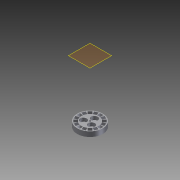
# Autodesk Inventor part: Bottom4
Saved by Autodesk Inventor 2012 (Build 160160000, 160)
## iProperties
Created: 2015-08-07
Part Number: Bottom4
Material: Default
Document SubType Name: Modeling
Designer: Craig
Density: 1 g/cm^3
Autodesk Inventor part; units mm, degrees
(part 1 of 3)
ref_plane "YZ Plane" through (0, 0, 0) normal (1, 0, 0) x (0, 1, 0)
ref_plane "XZ Plane" through (0, 0, 0) normal (0, 1, 0) x (-1, 0, 0)
ref_plane "XY Plane" through (0, 0, 0) normal (0, 0, 1) x (1, 0, 0)
sketch "BOTTOM" plane through (0, 0, 0) normal (0, 0, 1) x (1, 0, 0)
  line L0 (59.975, -52.845) -> (63.225, -52.845)
  line L1 (63.225, -52.845) -> (63.225, -49.595)
  line L2 (63.225, -49.595) -> (59.975, -49.595)
  line L3 (59.975, -49.595) -> (59.975, -52.845)
  line L4 (0, 0) -> (1, 0)
  line L5 (49.6005, -59.9784) -> (49.5995, -63.2284)
  line L6 (49.5995, -63.2284) -> (52.8495, -63.2295)
  line L7 (52.8495, -63.2295) -> (52.8505, -59.9795)
  line L8 (52.8505, -59.9795) -> (49.6005, -59.9784)
  line L9 (0, 0) -> (1, 0)
  line L10 (49.8915, -64.6991) -> (51.1369, -67.701)
  line L11 (51.1369, -67.701) -> (54.1388, -66.4556)
  line L12 (54.1388, -66.4556) -> (52.8934, -63.4537)
  line L13 (52.8934, -63.4537) -> (49.8915, -64.6991)
  line L14 (0, 0) -> (1, 0)
  line L15 (51.9695, -68.9456) -> (54.2706, -71.2407)
  line L16 (54.2706, -71.2407) -> (56.5657, -68.9397)
  line L17 (56.5657, -68.9397) -> (54.2646, -66.6445)
  line L18 (54.2646, -66.6445) -> (51.9695, -68.9456)
  line L19 (0, 0) -> (1, 0)
  line L20 (55.5107, -72.0693) -> (58.514, -73.3112)
  line L21 (58.514, -73.3112) -> (59.756, -70.3079)
  line L22 (59.756, -70.3079) -> (56.7527, -69.0659)
  line L23 (56.7527, -69.0659) -> (55.5107, -72.0693)
  line L24 (0, 0) -> (1, 0)
  line L25 (59.9813, -73.6029) -> (63.2313, -73.6008)
  line L26 (63.2313, -73.6008) -> (63.2293, -70.3508)
  line L27 (63.2293, -70.3508) -> (59.9793, -70.3529)
  line L28 (59.9793, -70.3529) -> (59.9813, -73.6029)
  line L29 (0, 0) -> (1, 0)
  line L30 (64.6994, -73.3084) -> (67.7011, -72.0624)
  line L31 (67.7011, -72.0624) -> (66.455, -69.0607)
  line L32 (66.455, -69.0607) -> (63.4534, -70.3067)
  line L33 (63.4534, -70.3067) -> (64.6994, -73.3084)
  line L34 (0, 0) -> (1, 0)
  line L35 (68.9435, -71.2317) -> (71.24, -68.932)
  line L36 (71.24, -68.932) -> (68.9403, -66.6355)
  line L37 (68.9403, -66.6355) -> (66.6438, -68.9351)
  line L38 (66.6438, -68.9351) -> (68.9435, -71.2317)
  line L39 (0, 0) -> (1, 0)
  line L40 (72.0699, -67.6893) -> (73.3118, -64.686)
  line L41 (73.3118, -64.686) -> (70.3085, -63.4441)
  line L42 (70.3085, -63.4441) -> (69.0665, -66.4474)
  line L43 (69.0665, -66.4474) -> (72.0699, -67.6893)
  line L44 (0, 0) -> (1, 0)
  line L45 (73.6037, -63.2169) -> (73.6013, -59.9669)
  line L46 (73.6013, -59.9669) -> (70.3513, -59.9694)
  line L47 (70.3513, -59.9694) -> (70.3537, -63.2194)
  line L48 (70.3537, -63.2194) -> (73.6037, -63.2169)
  line L49 (0, 0) -> (1, 0)
  line L50 (73.3095, -58.5022) -> (72.0634, -55.5006)
  line L51 (72.0634, -55.5006) -> (69.0618, -56.7467)
  line L52 (69.0618, -56.7467) -> (70.3079, -59.7483)
  line L53 (70.3079, -59.7483) -> (73.3095, -58.5022)
  line L54 (0, 0) -> (1, 0)
  line L55 (71.2319, -54.2571) -> (68.932, -51.9607)
  line L56 (68.932, -51.9607) -> (66.6357, -54.2606)
  line L57 (66.6357, -54.2606) -> (68.9355, -56.5569)
  line L58 (68.9355, -56.5569) -> (71.2319, -54.2571)
  line L59 (0, 0) -> (1, 0)
  line L60 (67.6871, -51.1295) -> (64.6835, -49.8882)
  line L61 (64.6835, -49.8882) -> (63.4422, -52.8918)
  line L62 (63.4422, -52.8918) -> (66.4458, -54.1331)
  line L63 (66.4458, -54.1331) -> (67.6871, -51.1295)
  line L64 (0, 0) -> (1, 0)
  line L65 (58.5019, -49.891) -> (55.5, -51.1366)
  line L66 (55.5, -51.1366) -> (56.7456, -54.1384)
  line L67 (56.7456, -54.1384) -> (59.7474, -52.8928)
  line L68 (59.7474, -52.8928) -> (58.5019, -49.891)
  line L69 (0, 0) -> (1, 0)
  line L70 (54.2559, -51.9683) -> (51.9595, -54.2681)
  line L71 (51.9595, -54.2681) -> (54.2593, -56.5645)
  line L72 (54.2593, -56.5645) -> (56.5557, -54.2647)
  line L73 (56.5557, -54.2647) -> (54.2559, -51.9683)
  line L74 (0, 0) -> (1, 0)
  line L75 (51.1301, -55.5101) -> (49.8882, -58.5135)
  line L76 (49.8882, -58.5135) -> (52.8916, -59.7554)
  line L77 (52.8916, -59.7554) -> (54.1334, -56.752)
  line L78 (54.1334, -56.752) -> (51.1301, -55.5101)
  line L79 (0, 0) -> (1, 0)
  arc A0 (48.6, -61.6029) -> (52.9038, -71.2653) centre (61.5843, -61.6091) ccw
  arc A1 (52.9038, -71.2653) -> (72.8082, -68.1903) centre (61.6004, -61.5999) ccw
  arc A2 (72.8082, -68.1903) -> (74.163, -58.2471) centre (61.5989, -61.5991) ccw
  arc A3 (74.163, -58.2471) -> (59.1805, -48.8249) centre (61.5986, -61.6031) ccw
  arc A4 (59.1805, -48.8249) -> (48.8055, -59.2842) centre (61.5989, -61.5991) ccw
  arc A5 (48.8055, -59.2842) -> (48.6, -61.6029) centre (61.5557, -61.583) ccw
  line L80 (0, 0) -> (1, 0)
  line L81 (55.9748, -59.9753) -> (56.0584, -59.9774)
  line L82 (56.0584, -59.9774) -> (56.141, -59.9837)
  line L83 (56.141, -59.9837) -> (56.2223, -59.994)
  line L84 (56.2223, -59.994) -> (56.3023, -60.0083)
  line L85 (56.3023, -60.0083) -> (56.3809, -60.0264)
  line L86 (56.3809, -60.0264) -> (56.458, -60.0483)
  line L87 (56.458, -60.0483) -> (56.5335, -60.0738)
  line L88 (56.5335, -60.0738) -> (56.6073, -60.1029)
  line L89 (56.6073, -60.1029) -> (56.6793, -60.1354)
  line L90 (56.6793, -60.1354) -> (56.7494, -60.1713)
  line L91 (56.7494, -60.1713) -> (56.8175, -60.2104)
  line L92 (56.8175, -60.2104) -> (56.8834, -60.2527)
  line L93 (56.8834, -60.2527) -> (56.9471, -60.298)
  line L94 (56.9471, -60.298) -> (57.0085, -60.3462)
  line L95 (57.0085, -60.3462) -> (57.0675, -60.3973)
  line L96 (57.0675, -60.3973) -> (57.1239, -60.4511)
  line L97 (57.1239, -60.4511) -> (57.1777, -60.5075)
  line L98 (57.1777, -60.5075) -> (57.2288, -60.5665)
  line L99 (57.2288, -60.5665) -> (57.2771, -60.6279)
  line L100 (57.2771, -60.6279) -> (57.3224, -60.6916)
  line L101 (57.3224, -60.6916) -> (57.3646, -60.7575)
  line L102 (57.3646, -60.7575) -> (57.4038, -60.8255)
  line L103 (57.4038, -60.8255) -> (57.4397, -60.8956)
  line L104 (57.4397, -60.8956) -> (57.4722, -60.9676)
  line L105 (57.4722, -60.9676) -> (57.5013, -61.0414)
  line L106 (57.5013, -61.0414) -> (57.5269, -61.1169)
  line L107 (57.5269, -61.1169) -> (57.5488, -61.194)
  line L108 (57.5488, -61.194) -> (57.5669, -61.2726)
  line L109 (57.5669, -61.2726) -> (57.5812, -61.3526)
  line L110 (57.5812, -61.3526) -> (57.5916, -61.4339)
  line L111 (57.5916, -61.4339) -> (57.5979, -61.5165)
  line L112 (57.5979, -61.5165) -> (57.6, -61.6001)
  line L113 (57.6, -61.6001) -> (57.5979, -61.6837)
  line L114 (57.5979, -61.6837) -> (57.5916, -61.7662)
  line L115 (57.5916, -61.7662) -> (57.5813, -61.8476)
  line L116 (57.5813, -61.8476) -> (57.567, -61.9276)
  line L117 (57.567, -61.9276) -> (57.5489, -62.0062)
  line L118 (57.5489, -62.0062) -> (57.527, -62.0833)
  line L119 (57.527, -62.0833) -> (57.5015, -62.1588)
  line L120 (57.5015, -62.1588) -> (57.4724, -62.2326)
  line L121 (57.4724, -62.2326) -> (57.4398, -62.3046)
  line L122 (57.4398, -62.3046) -> (57.404, -62.3747)
  line L123 (57.404, -62.3747) -> (57.3648, -62.4427)
  line L124 (57.3648, -62.4427) -> (57.3226, -62.5087)
  line L125 (57.3226, -62.5087) -> (57.2773, -62.5724)
  line L126 (57.2773, -62.5724) -> (57.2291, -62.6338)
  line L127 (57.2291, -62.6338) -> (57.178, -62.6928)
  line L128 (57.178, -62.6928) -> (57.1242, -62.7492)
  line L129 (57.1242, -62.7492) -> (57.0678, -62.803)
  line L130 (57.0678, -62.803) -> (57.0088, -62.8541)
  line L131 (57.0088, -62.8541) -> (56.9474, -62.9023)
  line L132 (56.9474, -62.9023) -> (56.8837, -62.9476)
  line L133 (56.8837, -62.9476) -> (56.8178, -62.9899)
  line L134 (56.8178, -62.9899) -> (56.7497, -63.0291)
  line L135 (56.7497, -63.0291) -> (56.6797, -63.065)
  line L136 (56.6797, -63.065) -> (56.6077, -63.0975)
  line L137 (56.6077, -63.0975) -> (56.5339, -63.1266)
  line L138 (56.5339, -63.1266) -> (56.4584, -63.1522)
  line L139 (56.4584, -63.1522) -> (56.3813, -63.1741)
  line L140 (56.3813, -63.1741) -> (56.3027, -63.1922)
  line L141 (56.3027, -63.1922) -> (56.2227, -63.2065)
  line L142 (56.2227, -63.2065) -> (56.1413, -63.2169)
  line L143 (56.1413, -63.2169) -> (56.0588, -63.2232)
  line L144 (56.0588, -63.2232) -> (55.9752, -63.2253)
  line L145 (55.9752, -63.2253) -> (55.8916, -63.2232)
  line L146 (55.8916, -63.2232) -> (55.809, -63.2169)
  line L147 (55.809, -63.2169) -> (55.7277, -63.2066)
  line L148 (55.7277, -63.2066) -> (55.6477, -63.1923)
  line L149 (55.6477, -63.1923) -> (55.5691, -63.1742)
  line L150 (55.5691, -63.1742) -> (55.492, -63.1523)
  line L151 (55.492, -63.1523) -> (55.4165, -63.1267)
  line L152 (55.4165, -63.1267) -> (55.3427, -63.0977)
  line L153 (55.3427, -63.0977) -> (55.2707, -63.0651)
  line L154 (55.2707, -63.0651) -> (55.2006, -63.0292)
  line L155 (55.2006, -63.0292) -> (55.1325, -62.9901)
  line L156 (55.1325, -62.9901) -> (55.0666, -62.9479)
  line L157 (55.0666, -62.9479) -> (55.0029, -62.9026)
  line L158 (55.0029, -62.9026) -> (54.9415, -62.8543)
  line L159 (54.9415, -62.8543) -> (54.8825, -62.8033)
  line L160 (54.8825, -62.8033) -> (54.8261, -62.7495)
  line L161 (54.8261, -62.7495) -> (54.7723, -62.693)
  line L162 (54.7723, -62.693) -> (54.7212, -62.6341)
  line L163 (54.7212, -62.6341) -> (54.6729, -62.5727)
  line L164 (54.6729, -62.5727) -> (54.6276, -62.509)
  line L165 (54.6276, -62.509) -> (54.5854, -62.4431)
  line L166 (54.5854, -62.4431) -> (54.5462, -62.375)
  line L167 (54.5462, -62.375) -> (54.5103, -62.305)
  line L168 (54.5103, -62.305) -> (54.4778, -62.233)
  line L169 (54.4778, -62.233) -> (54.4487, -62.1592)
  line L170 (54.4487, -62.1592) -> (54.4231, -62.0837)
  line L171 (54.4231, -62.0837) -> (54.4012, -62.0066)
  line L172 (54.4012, -62.0066) -> (54.3831, -61.928)
  line L173 (54.3831, -61.928) -> (54.3688, -61.8479)
  line L174 (54.3688, -61.8479) -> (54.3584, -61.7666)
  line L175 (54.3584, -61.7666) -> (54.3521, -61.6841)
  line L176 (54.3521, -61.6841) -> (54.35, -61.6005)
  line L177 (54.35, -61.6005) -> (54.3521, -61.5169)
  line L178 (54.3521, -61.5169) -> (54.3584, -61.4343)
  line L179 (54.3584, -61.4343) -> (54.3687, -61.353)
  line L180 (54.3687, -61.353) -> (54.383, -61.273)
  line L181 (54.383, -61.273) -> (54.4011, -61.1944)
  line L182 (54.4011, -61.1944) -> (54.423, -61.1172)
  line L183 (54.423, -61.1172) -> (54.4485, -61.0417)
  line L184 (54.4485, -61.0417) -> (54.4776, -60.9679)
  line L185 (54.4776, -60.9679) -> (54.5102, -60.8959)
  line L186 (54.5102, -60.8959) -> (54.546, -60.8259)
  line L187 (54.546, -60.8259) -> (54.5852, -60.7578)
  line L188 (54.5852, -60.7578) -> (54.6274, -60.6919)
  line L189 (54.6274, -60.6919) -> (54.6727, -60.6282)
  line L190 (54.6727, -60.6282) -> (54.7209, -60.5668)
  line L191 (54.7209, -60.5668) -> (54.772, -60.5078)
  line L192 (54.772, -60.5078) -> (54.8258, -60.4514)
  line L193 (54.8258, -60.4514) -> (54.8822, -60.3976)
  line L194 (54.8822, -60.3976) -> (54.9412, -60.3465)
  line L195 (54.9412, -60.3465) -> (55.0026, -60.2982)
  line L196 (55.0026, -60.2982) -> (55.0663, -60.2529)
  line L197 (55.0663, -60.2529) -> (55.1322, -60.2106)
  line L198 (55.1322, -60.2106) -> (55.2003, -60.1715)
  line L199 (55.2003, -60.1715) -> (55.2703, -60.1356)
  line L200 (55.2703, -60.1356) -> (55.3423, -60.1031)
  line L201 (55.3423, -60.1031) -> (55.4161, -60.074)
  line L202 (55.4161, -60.074) -> (55.4916, -60.0484)
  line L203 (55.4916, -60.0484) -> (55.5687, -60.0265)
  line L204 (55.5687, -60.0265) -> (55.6473, -60.0083)
  line L205 (55.6473, -60.0083) -> (55.7273, -59.994)
  line L206 (55.7273, -59.994) -> (55.8087, -59.9837)
  line L207 (55.8087, -59.9837) -> (55.8912, -59.9774)
  line L208 (55.8912, -59.9774) -> (55.9748, -59.9753)
  line L209 (0, 0) -> (1, 0)
  line L210 (59.977, -67.2264) -> (59.9791, -67.1428)
  line L211 (59.9791, -67.1428) -> (59.9853, -67.0602)
  line L212 (59.9853, -67.0602) -> (59.9956, -66.9789)
  line L213 (59.9956, -66.9789) -> (60.0099, -66.8989)
  line L214 (60.0099, -66.8989) -> (60.028, -66.8202)
  line L215 (60.028, -66.8202) -> (60.0498, -66.7431)
  line L216 (60.0498, -66.7431) -> (60.0754, -66.6676)
  line L217 (60.0754, -66.6676) -> (60.1044, -66.5938)
  line L218 (60.1044, -66.5938) -> (60.1369, -66.5218)
  line L219 (60.1369, -66.5218) -> (60.1728, -66.4517)
  line L220 (60.1728, -66.4517) -> (60.2119, -66.3837)
  line L221 (60.2119, -66.3837) -> (60.2541, -66.3177)
  line L222 (60.2541, -66.3177) -> (60.2994, -66.254)
  line L223 (60.2994, -66.254) -> (60.3476, -66.1926)
  line L224 (60.3476, -66.1926) -> (60.3987, -66.1336)
  line L225 (60.3987, -66.1336) -> (60.4524, -66.0771)
  line L226 (60.4524, -66.0771) -> (60.5088, -66.0233)
  line L227 (60.5088, -66.0233) -> (60.5678, -65.9722)
  line L228 (60.5678, -65.9722) -> (60.6291, -65.9239)
  line L229 (60.6291, -65.9239) -> (60.6928, -65.8786)
  line L230 (60.6928, -65.8786) -> (60.7587, -65.8363)
  line L231 (60.7587, -65.8363) -> (60.8268, -65.7971)
  line L232 (60.8268, -65.7971) -> (60.8968, -65.7612)
  line L233 (60.8968, -65.7612) -> (60.9688, -65.7286)
  line L234 (60.9688, -65.7286) -> (61.0426, -65.6995)
  line L235 (61.0426, -65.6995) -> (61.1181, -65.6739)
  line L236 (61.1181, -65.6739) -> (61.1952, -65.652)
  line L237 (61.1952, -65.652) -> (61.2738, -65.6338)
  line L238 (61.2738, -65.6338) -> (61.3538, -65.6195)
  line L239 (61.3538, -65.6195) -> (61.4351, -65.6091)
  line L240 (61.4351, -65.6091) -> (61.5176, -65.6028)
  line L241 (61.5176, -65.6028) -> (61.6013, -65.6006)
  line L242 (61.6013, -65.6006) -> (61.6849, -65.6027)
  line L243 (61.6849, -65.6027) -> (61.7674, -65.609)
  line L244 (61.7674, -65.609) -> (61.8487, -65.6193)
  line L245 (61.8487, -65.6193) -> (61.9288, -65.6335)
  line L246 (61.9288, -65.6335) -> (62.0074, -65.6516)
  line L247 (62.0074, -65.6516) -> (62.0845, -65.6735)
  line L248 (62.0845, -65.6735) -> (62.16, -65.699)
  line L249 (62.16, -65.699) -> (62.2338, -65.7281)
  line L250 (62.2338, -65.7281) -> (62.3058, -65.7606)
  line L251 (62.3058, -65.7606) -> (62.3759, -65.7964)
  line L252 (62.3759, -65.7964) -> (62.444, -65.8355)
  line L253 (62.444, -65.8355) -> (62.5099, -65.8777)
  line L254 (62.5099, -65.8777) -> (62.5737, -65.923)
  line L255 (62.5737, -65.923) -> (62.6351, -65.9712)
  line L256 (62.6351, -65.9712) -> (62.6941, -66.0223)
  line L257 (62.6941, -66.0223) -> (62.7505, -66.0761)
  line L258 (62.7505, -66.0761) -> (62.8044, -66.1325)
  line L259 (62.8044, -66.1325) -> (62.8555, -66.1914)
  line L260 (62.8555, -66.1914) -> (62.9037, -66.2528)
  line L261 (62.9037, -66.2528) -> (62.9491, -66.3165)
  line L262 (62.9491, -66.3165) -> (62.9914, -66.3824)
  line L263 (62.9914, -66.3824) -> (63.0305, -66.4504)
  line L264 (63.0305, -66.4504) -> (63.0664, -66.5205)
  line L265 (63.0664, -66.5205) -> (63.099, -66.5924)
  line L266 (63.099, -66.5924) -> (63.1281, -66.6662)
  line L267 (63.1281, -66.6662) -> (63.1537, -66.7417)
  line L268 (63.1537, -66.7417) -> (63.1757, -66.8188)
  line L269 (63.1757, -66.8188) -> (63.1938, -66.8974)
  line L270 (63.1938, -66.8974) -> (63.2082, -66.9774)
  line L271 (63.2082, -66.9774) -> (63.2185, -67.0588)
  line L272 (63.2185, -67.0588) -> (63.2249, -67.1413)
  line L273 (63.2249, -67.1413) -> (63.227, -67.2249)
  line L274 (63.227, -67.2249) -> (63.2249, -67.3085)
  line L275 (63.2249, -67.3085) -> (63.2187, -67.391)
  line L276 (63.2187, -67.391) -> (63.2084, -67.4724)
  line L277 (63.2084, -67.4724) -> (63.1941, -67.5524)
  line L278 (63.1941, -67.5524) -> (63.176, -67.631)
  line L279 (63.176, -67.631) -> (63.1542, -67.7082)
  line L280 (63.1542, -67.7082) -> (63.1287, -67.7837)
  line L281 (63.1287, -67.7837) -> (63.0996, -67.8575)
  line L282 (63.0996, -67.8575) -> (63.0671, -67.9295)
  line L283 (63.0671, -67.9295) -> (63.0312, -67.9996)
  line L284 (63.0312, -67.9996) -> (62.9921, -68.0676)
  line L285 (62.9921, -68.0676) -> (62.9499, -68.1336)
  line L286 (62.9499, -68.1336) -> (62.9046, -68.1973)
  line L287 (62.9046, -68.1973) -> (62.8564, -68.2587)
  line L288 (62.8564, -68.2587) -> (62.8054, -68.3177)
  line L289 (62.8054, -68.3177) -> (62.7516, -68.3742)
  line L290 (62.7516, -68.3742) -> (62.6952, -68.428)
  line L291 (62.6952, -68.428) -> (62.6362, -68.4791)
  line L292 (62.6362, -68.4791) -> (62.5749, -68.5274)
  line L293 (62.5749, -68.5274) -> (62.5112, -68.5727)
  line L294 (62.5112, -68.5727) -> (62.4453, -68.615)
  line L295 (62.4453, -68.615) -> (62.3772, -68.6542)
  line L296 (62.3772, -68.6542) -> (62.3072, -68.6901)
  line L297 (62.3072, -68.6901) -> (62.2352, -68.7226)
  line L298 (62.2352, -68.7226) -> (62.1614, -68.7518)
  line L299 (62.1614, -68.7518) -> (62.0859, -68.7774)
  line L300 (62.0859, -68.7774) -> (62.0088, -68.7993)
  line L301 (62.0088, -68.7993) -> (61.9302, -68.8175)
  line L302 (61.9302, -68.8175) -> (61.8502, -68.8318)
  line L303 (61.8502, -68.8318) -> (61.7689, -68.8422)
  line L304 (61.7689, -68.8422) -> (61.6864, -68.8485)
  line L305 (61.6864, -68.8485) -> (61.6028, -68.8506)
  line L306 (61.6028, -68.8506) -> (61.5191, -68.8486)
  line L307 (61.5191, -68.8486) -> (61.4366, -68.8423)
  line L308 (61.4366, -68.8423) -> (61.3553, -68.832)
  line L309 (61.3553, -68.832) -> (61.2752, -68.8178)
  line L310 (61.2752, -68.8178) -> (61.1966, -68.7997)
  line L311 (61.1966, -68.7997) -> (61.1195, -68.7778)
  line L312 (61.1195, -68.7778) -> (61.044, -68.7523)
  line L313 (61.044, -68.7523) -> (60.9702, -68.7232)
  line L314 (60.9702, -68.7232) -> (60.8982, -68.6907)
  line L315 (60.8982, -68.6907) -> (60.8281, -68.6549)
  line L316 (60.8281, -68.6549) -> (60.76, -68.6158)
  line L317 (60.76, -68.6158) -> (60.6941, -68.5735)
  line L318 (60.6941, -68.5735) -> (60.6303, -68.5283)
  line L319 (60.6303, -68.5283) -> (60.5689, -68.48)
  line L320 (60.5689, -68.48) -> (60.5099, -68.429)
  line L321 (60.5099, -68.429) -> (60.4535, -68.3752)
  line L322 (60.4535, -68.3752) -> (60.3997, -68.3188)
  line L323 (60.3997, -68.3188) -> (60.3486, -68.2599)
  line L324 (60.3486, -68.2599) -> (60.3003, -68.1985)
  line L325 (60.3003, -68.1985) -> (60.2549, -68.1348)
  line L326 (60.2549, -68.1348) -> (60.2126, -68.0689)
  line L327 (60.2126, -68.0689) -> (60.1735, -68.0009)
  line L328 (60.1735, -68.0009) -> (60.1376, -67.9308)
  line L329 (60.1376, -67.9308) -> (60.105, -67.8588)
  line L330 (60.105, -67.8588) -> (60.0759, -67.7851)
  line L331 (60.0759, -67.7851) -> (60.0503, -67.7096)
  line L332 (60.0503, -67.7096) -> (60.0284, -67.6325)
  line L333 (60.0284, -67.6325) -> (60.0102, -67.5539)
  line L334 (60.0102, -67.5539) -> (59.9958, -67.4738)
  line L335 (59.9958, -67.4738) -> (59.9855, -67.3925)
  line L336 (59.9855, -67.3925) -> (59.9792, -67.31)
  line L337 (59.9792, -67.31) -> (59.977, -67.2264)
  line L338 (0, 0) -> (1, 0)
  line L339 (67.2261, -63.2233) -> (67.1425, -63.2212)
  line L340 (67.1425, -63.2212) -> (67.06, -63.215)
  line L341 (67.06, -63.215) -> (66.9786, -63.2047)
  line L342 (66.9786, -63.2047) -> (66.8986, -63.1904)
  line L343 (66.8986, -63.1904) -> (66.82, -63.1723)
  line L344 (66.82, -63.1723) -> (66.7429, -63.1504)
  line L345 (66.7429, -63.1504) -> (66.6673, -63.1249)
  line L346 (66.6673, -63.1249) -> (66.5935, -63.0959)
  line L347 (66.5935, -63.0959) -> (66.5215, -63.0633)
  line L348 (66.5215, -63.0633) -> (66.4515, -63.0275)
  line L349 (66.4515, -63.0275) -> (66.3834, -62.9884)
  line L350 (66.3834, -62.9884) -> (66.3174, -62.9461)
  line L351 (66.3174, -62.9461) -> (66.2537, -62.9009)
  line L352 (66.2537, -62.9009) -> (66.1923, -62.8526)
  line L353 (66.1923, -62.8526) -> (66.1333, -62.8016)
  line L354 (66.1333, -62.8016) -> (66.0769, -62.7478)
  line L355 (66.0769, -62.7478) -> (66.023, -62.6914)
  line L356 (66.023, -62.6914) -> (65.9719, -62.6325)
  line L357 (65.9719, -62.6325) -> (65.9237, -62.5711)
  line L358 (65.9237, -62.5711) -> (65.8783, -62.5074)
  line L359 (65.8783, -62.5074) -> (65.8361, -62.4415)
  line L360 (65.8361, -62.4415) -> (65.7969, -62.3734)
  line L361 (65.7969, -62.3734) -> (65.761, -62.3034)
  line L362 (65.761, -62.3034) -> (65.7284, -62.2314)
  line L363 (65.7284, -62.2314) -> (65.6993, -62.1576)
  line L364 (65.6993, -62.1576) -> (65.6737, -62.0821)
  line L365 (65.6737, -62.0821) -> (65.6518, -62.005)
  line L366 (65.6518, -62.005) -> (65.6336, -61.9264)
  line L367 (65.6336, -61.9264) -> (65.6193, -61.8464)
  line L368 (65.6193, -61.8464) -> (65.6089, -61.7651)
  line L369 (65.6089, -61.7651) -> (65.6026, -61.6826)
  line L370 (65.6026, -61.6826) -> (65.6005, -61.599)
  line L371 (65.6005, -61.599) -> (65.6025, -61.5153)
  line L372 (65.6025, -61.5153) -> (65.6088, -61.4328)
  line L373 (65.6088, -61.4328) -> (65.6191, -61.3515)
  line L374 (65.6191, -61.3515) -> (65.6333, -61.2714)
  line L375 (65.6333, -61.2714) -> (65.6515, -61.1928)
  line L376 (65.6515, -61.1928) -> (65.6733, -61.1157)
  line L377 (65.6733, -61.1157) -> (65.6988, -61.0402)
  line L378 (65.6988, -61.0402) -> (65.7279, -60.9664)
  line L379 (65.7279, -60.9664) -> (65.7604, -60.8944)
  line L380 (65.7604, -60.8944) -> (65.7963, -60.8243)
  line L381 (65.7963, -60.8243) -> (65.8354, -60.7562)
  line L382 (65.8354, -60.7562) -> (65.8776, -60.6903)
  line L383 (65.8776, -60.6903) -> (65.9229, -60.6266)
  line L384 (65.9229, -60.6266) -> (65.9711, -60.5652)
  line L385 (65.9711, -60.5652) -> (66.0222, -60.5062)
  line L386 (66.0222, -60.5062) -> (66.0759, -60.4497)
  line L387 (66.0759, -60.4497) -> (66.1324, -60.3959)
  line L388 (66.1324, -60.3959) -> (66.1913, -60.3448)
  line L389 (66.1913, -60.3448) -> (66.2527, -60.2965)
  line L390 (66.2527, -60.2965) -> (66.3164, -60.2512)
  line L391 (66.3164, -60.2512) -> (66.3823, -60.2089)
  line L392 (66.3823, -60.2089) -> (66.4503, -60.1697)
  line L393 (66.4503, -60.1697) -> (66.5204, -60.1338)
  line L394 (66.5204, -60.1338) -> (66.5923, -60.1013)
  line L395 (66.5923, -60.1013) -> (66.6661, -60.0721)
  line L396 (66.6661, -60.0721) -> (66.7416, -60.0465)
  line L397 (66.7416, -60.0465) -> (66.8187, -60.0246)
  line L398 (66.8187, -60.0246) -> (66.8973, -60.0064)
  line L399 (66.8973, -60.0064) -> (66.9773, -59.9921)
  line L400 (66.9773, -59.9921) -> (67.0587, -59.9818)
  line L401 (67.0587, -59.9818) -> (67.1412, -59.9754)
  line L402 (67.1412, -59.9754) -> (67.2248, -59.9733)
  line L403 (67.2248, -59.9733) -> (67.3084, -59.9754)
  line L404 (67.3084, -59.9754) -> (67.391, -59.9816)
  line L405 (67.391, -59.9816) -> (67.4723, -59.9919)
  line L406 (67.4723, -59.9919) -> (67.5523, -60.0062)
  line L407 (67.5523, -60.0062) -> (67.6309, -60.0243)
  line L408 (67.6309, -60.0243) -> (67.7081, -60.0462)
  line L409 (67.7081, -60.0462) -> (67.7836, -60.0717)
  line L410 (67.7836, -60.0717) -> (67.8574, -60.1007)
  line L411 (67.8574, -60.1007) -> (67.9294, -60.1333)
  line L412 (67.9294, -60.1333) -> (67.9995, -60.1691)
  line L413 (67.9995, -60.1691) -> (68.0675, -60.2082)
  line L414 (68.0675, -60.2082) -> (68.1335, -60.2505)
  line L415 (68.1335, -60.2505) -> (68.1972, -60.2957)
  line L416 (68.1972, -60.2957) -> (68.2586, -60.344)
  line L417 (68.2586, -60.344) -> (68.3176, -60.395)
  line L418 (68.3176, -60.395) -> (68.374, -60.4488)
  line L419 (68.374, -60.4488) -> (68.4279, -60.5052)
  line L420 (68.4279, -60.5052) -> (68.479, -60.5641)
  line L421 (68.479, -60.5641) -> (68.5272, -60.6255)
  line L422 (68.5272, -60.6255) -> (68.5726, -60.6892)
  line L423 (68.5726, -60.6892) -> (68.6149, -60.7551)
  line L424 (68.6149, -60.7551) -> (68.654, -60.8232)
  line L425 (68.654, -60.8232) -> (68.6899, -60.8932)
  line L426 (68.6899, -60.8932) -> (68.7225, -60.9652)
  line L427 (68.7225, -60.9652) -> (68.7516, -61.039)
  line L428 (68.7516, -61.039) -> (68.7772, -61.1144)
  line L429 (68.7772, -61.1144) -> (68.7991, -61.1916)
  line L430 (68.7991, -61.1916) -> (68.8173, -61.2702)
  line L431 (68.8173, -61.2702) -> (68.8316, -61.3502)
  line L432 (68.8316, -61.3502) -> (68.842, -61.4315)
  line L433 (68.842, -61.4315) -> (68.8483, -61.514)
  line L434 (68.8483, -61.514) -> (68.8505, -61.5976)
  line L435 (68.8505, -61.5976) -> (68.8484, -61.6813)
  line L436 (68.8484, -61.6813) -> (68.8421, -61.7638)
  line L437 (68.8421, -61.7638) -> (68.8318, -61.8451)
  line L438 (68.8318, -61.8451) -> (68.8176, -61.9252)
  line L439 (68.8176, -61.9252) -> (68.7995, -62.0038)
  line L440 (68.7995, -62.0038) -> (68.7776, -62.0809)
  line L441 (68.7776, -62.0809) -> (68.7521, -62.1564)
  line L442 (68.7521, -62.1564) -> (68.723, -62.2302)
  line L443 (68.723, -62.2302) -> (68.6905, -62.3022)
  line L444 (68.6905, -62.3022) -> (68.6546, -62.3723)
  line L445 (68.6546, -62.3723) -> (68.6155, -62.4404)
  line L446 (68.6155, -62.4404) -> (68.5733, -62.5063)
  line L447 (68.5733, -62.5063) -> (68.528, -62.57)
  line L448 (68.528, -62.57) -> (68.4798, -62.6314)
  line L449 (68.4798, -62.6314) -> (68.4288, -62.6904)
  line L450 (68.4288, -62.6904) -> (68.375, -62.7469)
  line L451 (68.375, -62.7469) -> (68.3186, -62.8007)
  line L452 (68.3186, -62.8007) -> (68.2596, -62.8518)
  line L453 (68.2596, -62.8518) -> (68.1982, -62.9001)
  line L454 (68.1982, -62.9001) -> (68.1346, -62.9454)
  line L455 (68.1346, -62.9454) -> (68.0686, -62.9877)
  line L456 (68.0686, -62.9877) -> (68.0006, -63.0269)
  line L457 (68.0006, -63.0269) -> (67.9306, -63.0628)
  line L458 (67.9306, -63.0628) -> (67.8586, -63.0953)
  line L459 (67.8586, -63.0953) -> (67.7848, -63.1245)
  line L460 (67.7848, -63.1245) -> (67.7093, -63.15)
  line L461 (67.7093, -63.15) -> (67.6322, -63.172)
  line L462 (67.6322, -63.172) -> (67.5536, -63.1902)
  line L463 (67.5536, -63.1902) -> (67.4736, -63.2045)
  line L464 (67.4736, -63.2045) -> (67.3923, -63.2148)
  line L465 (67.3923, -63.2148) -> (67.3097, -63.2211)
  line L466 (67.3097, -63.2211) -> (67.2261, -63.2233)
  line L467 (0, 0) -> (1, 0)
  line L468 (63.2244, -55.9741) -> (63.2223, -56.0577)
  line L469 (63.2223, -56.0577) -> (63.2161, -56.1402)
  line L470 (63.2161, -56.1402) -> (63.2058, -56.2215)
  line L471 (63.2058, -56.2215) -> (63.1915, -56.3016)
  line L472 (63.1915, -56.3016) -> (63.1734, -56.3802)
  line L473 (63.1734, -56.3802) -> (63.1515, -56.4573)
  line L474 (63.1515, -56.4573) -> (63.126, -56.5328)
  line L475 (63.126, -56.5328) -> (63.0969, -56.6066)
  line L476 (63.0969, -56.6066) -> (63.0644, -56.6786)
  line L477 (63.0644, -56.6786) -> (63.0285, -56.7487)
  line L478 (63.0285, -56.7487) -> (62.9894, -56.8167)
  line L479 (62.9894, -56.8167) -> (62.9472, -56.8827)
  line L480 (62.9472, -56.8827) -> (62.9019, -56.9464)
  line L481 (62.9019, -56.9464) -> (62.8537, -57.0078)
  line L482 (62.8537, -57.0078) -> (62.8026, -57.0668)
  line L483 (62.8026, -57.0668) -> (62.7488, -57.1232)
  line L484 (62.7488, -57.1232) -> (62.6924, -57.1771)
  line L485 (62.6924, -57.1771) -> (62.6334, -57.2282)
  line L486 (62.6334, -57.2282) -> (62.5721, -57.2764)
  line L487 (62.5721, -57.2764) -> (62.5084, -57.3217)
  line L488 (62.5084, -57.3217) -> (62.4424, -57.364)
  line L489 (62.4424, -57.364) -> (62.3744, -57.4032)
  line L490 (62.3744, -57.4032) -> (62.3044, -57.4391)
  line L491 (62.3044, -57.4391) -> (62.2324, -57.4716)
  line L492 (62.2324, -57.4716) -> (62.1586, -57.5008)
  line L493 (62.1586, -57.5008) -> (62.0831, -57.5263)
  line L494 (62.0831, -57.5263) -> (62.006, -57.5482)
  line L495 (62.006, -57.5482) -> (61.9274, -57.5664)
  line L496 (61.9274, -57.5664) -> (61.8474, -57.5807)
  line L497 (61.8474, -57.5807) -> (61.766, -57.5911)
  line L498 (61.766, -57.5911) -> (61.6835, -57.5974)
  line L499 (61.6835, -57.5974) -> (61.5999, -57.5995)
  line L500 (61.5999, -57.5995) -> (61.5163, -57.5974)
  line L501 (61.5163, -57.5974) -> (61.4337, -57.5912)
  line L502 (61.4337, -57.5912) -> (61.3524, -57.5809)
  line L503 (61.3524, -57.5809) -> (61.2724, -57.5666)
  line L504 (61.2724, -57.5666) -> (61.1938, -57.5485)
  line L505 (61.1938, -57.5485) -> (61.1166, -57.5266)
  line L506 (61.1166, -57.5266) -> (61.0411, -57.5011)
  line L507 (61.0411, -57.5011) -> (60.9673, -57.472)
  line L508 (60.9673, -57.472) -> (60.8953, -57.4395)
  line L509 (60.8953, -57.4395) -> (60.8253, -57.4036)
  line L510 (60.8253, -57.4036) -> (60.7572, -57.3645)
  line L511 (60.7572, -57.3645) -> (60.6913, -57.3222)
  line L512 (60.6913, -57.3222) -> (60.6275, -57.277)
  line L513 (60.6275, -57.277) -> (60.5661, -57.2287)
  line L514 (60.5661, -57.2287) -> (60.5072, -57.1777)
  line L515 (60.5072, -57.1777) -> (60.4507, -57.1239)
  line L516 (60.4507, -57.1239) -> (60.3969, -57.0675)
  line L517 (60.3969, -57.0675) -> (60.3458, -57.0085)
  line L518 (60.3458, -57.0085) -> (60.2975, -56.9471)
  line L519 (60.2975, -56.9471) -> (60.2522, -56.8834)
  line L520 (60.2522, -56.8834) -> (60.2099, -56.8175)
  line L521 (60.2099, -56.8175) -> (60.1708, -56.7495)
  line L522 (60.1708, -56.7495) -> (60.1349, -56.6794)
  line L523 (60.1349, -56.6794) -> (60.1023, -56.6075)
  line L524 (60.1023, -56.6075) -> (60.0732, -56.5337)
  line L525 (60.0732, -56.5337) -> (60.0476, -56.4582)
  line L526 (60.0476, -56.4582) -> (60.0257, -56.3811)
  line L527 (60.0257, -56.3811) -> (60.0075, -56.3025)
  line L528 (60.0075, -56.3025) -> (59.9932, -56.2224)
  line L529 (59.9932, -56.2224) -> (59.9829, -56.1411)
  line L530 (59.9829, -56.1411) -> (59.9766, -56.0586)
  line L531 (59.9766, -56.0586) -> (59.9744, -55.975)
  line L532 (59.9744, -55.975) -> (59.9765, -55.8914)
  line L533 (59.9765, -55.8914) -> (59.9828, -55.8088)
  line L534 (59.9828, -55.8088) -> (59.9931, -55.7275)
  line L535 (59.9931, -55.7275) -> (60.0074, -55.6475)
  line L536 (60.0074, -55.6475) -> (60.0255, -55.5688)
  line L537 (60.0255, -55.5688) -> (60.0474, -55.4917)
  line L538 (60.0474, -55.4917) -> (60.0729, -55.4162)
  line L539 (60.0729, -55.4162) -> (60.102, -55.3424)
  line L540 (60.102, -55.3424) -> (60.1345, -55.2704)
  line L541 (60.1345, -55.2704) -> (60.1703, -55.2003)
  line L542 (60.1703, -55.2003) -> (60.2095, -55.1323)
  line L543 (60.2095, -55.1323) -> (60.2517, -55.0663)
  line L544 (60.2517, -55.0663) -> (60.297, -55.0026)
  line L545 (60.297, -55.0026) -> (60.3452, -54.9412)
  line L546 (60.3452, -54.9412) -> (60.3963, -54.8822)
  line L547 (60.3963, -54.8822) -> (60.4501, -54.8258)
  line L548 (60.4501, -54.8258) -> (60.5065, -54.772)
  line L549 (60.5065, -54.772) -> (60.5654, -54.7209)
  line L550 (60.5654, -54.7209) -> (60.6268, -54.6726)
  line L551 (60.6268, -54.6726) -> (60.6905, -54.6273)
  line L552 (60.6905, -54.6273) -> (60.7564, -54.585)
  line L553 (60.7564, -54.585) -> (60.8245, -54.5459)
  line L554 (60.8245, -54.5459) -> (60.8945, -54.51)
  line L555 (60.8945, -54.51) -> (60.9665, -54.4774)
  line L556 (60.9665, -54.4774) -> (61.0403, -54.4483)
  line L557 (61.0403, -54.4483) -> (61.1158, -54.4227)
  line L558 (61.1158, -54.4227) -> (61.1929, -54.4008)
  line L559 (61.1929, -54.4008) -> (61.2715, -54.3826)
  line L560 (61.2715, -54.3826) -> (61.3515, -54.3683)
  line L561 (61.3515, -54.3683) -> (61.4328, -54.358)
  line L562 (61.4328, -54.358) -> (61.5154, -54.3517)
  line L563 (61.5154, -54.3517) -> (61.599, -54.3495)
  line L564 (61.599, -54.3495) -> (61.6826, -54.3516)
  line L565 (61.6826, -54.3516) -> (61.7651, -54.3579)
  line L566 (61.7651, -54.3579) -> (61.8465, -54.3682)
  line L567 (61.8465, -54.3682) -> (61.9265, -54.3824)
  line L568 (61.9265, -54.3824) -> (62.0051, -54.4006)
  line L569 (62.0051, -54.4006) -> (62.0822, -54.4224)
  line L570 (62.0822, -54.4224) -> (62.1577, -54.448)
  line L571 (62.1577, -54.448) -> (62.2315, -54.477)
  line L572 (62.2315, -54.477) -> (62.3035, -54.5096)
  line L573 (62.3035, -54.5096) -> (62.3736, -54.5454)
  line L574 (62.3736, -54.5454) -> (62.4417, -54.5845)
  line L575 (62.4417, -54.5845) -> (62.5076, -54.6268)
  line L576 (62.5076, -54.6268) -> (62.5713, -54.6721)
  line L577 (62.5713, -54.6721) -> (62.6327, -54.7203)
  line L578 (62.6327, -54.7203) -> (62.6917, -54.7714)
  line L579 (62.6917, -54.7714) -> (62.7482, -54.8251)
  line L580 (62.7482, -54.8251) -> (62.802, -54.8816)
  line L581 (62.802, -54.8816) -> (62.8531, -54.9405)
  line L582 (62.8531, -54.9405) -> (62.9013, -55.0019)
  line L583 (62.9013, -55.0019) -> (62.9467, -55.0656)
  line L584 (62.9467, -55.0656) -> (62.9889, -55.1315)
  line L585 (62.9889, -55.1315) -> (63.0281, -55.1995)
  line L586 (63.0281, -55.1995) -> (63.064, -55.2696)
  line L587 (63.064, -55.2696) -> (63.0966, -55.3416)
  line L588 (63.0966, -55.3416) -> (63.1257, -55.4154)
  line L589 (63.1257, -55.4154) -> (63.1512, -55.4909)
  line L590 (63.1512, -55.4909) -> (63.1732, -55.568)
  line L591 (63.1732, -55.568) -> (63.1913, -55.6466)
  line L592 (63.1913, -55.6466) -> (63.2056, -55.7266)
  line L593 (63.2056, -55.7266) -> (63.216, -55.8079)
  line L594 (63.216, -55.8079) -> (63.2223, -55.8904)
  line L595 (63.2223, -55.8904) -> (63.2244, -55.9741)
  line L596 (0, 0) -> (1, 0)
  constraints: 1194 end point, 12 point on circle, 6 centre point
extrude "Extrusion1" add sketch "BOTTOM" along normal blind 4
sketch "Sketch4" plane through (0, 0, 0) normal (0, 0, -1) x (-1, 0, 0)
  line L0 (-59.975, -49.595) -> (-59.975, -52.845) projected
  line L1 (-59.975, -52.845) -> (-63.225, -52.845) projected
  line L2 (-63.225, -52.845) -> (-63.225, -49.595) projected
  line L3 (-63.225, -49.595) -> (-59.975, -49.595) projected
  line L4 (-52.8934, -63.4537) -> (-49.8915, -64.6991) projected
  line L5 (-49.8915, -64.6991) -> (-51.1369, -67.701) projected
  line L6 (-51.1369, -67.701) -> (-54.1388, -66.4556) projected
  line L7 (-54.1388, -66.4556) -> (-52.8934, -63.4537) projected
  line L8 (-54.2646, -66.6445) -> (-51.9695, -68.9456) projected
  line L9 (-51.9695, -68.9456) -> (-54.2706, -71.2407) projected
  line L10 (-54.2706, -71.2407) -> (-56.5657, -68.9397) projected
  line L11 (-56.5657, -68.9397) -> (-54.2646, -66.6445) projected
  line L12 (-56.7527, -69.0659) -> (-55.5107, -72.0693) projected
  line L13 (-55.5107, -72.0693) -> (-58.514, -73.3112) projected
  line L14 (-58.514, -73.3112) -> (-59.756, -70.3079) projected
  line L15 (-59.756, -70.3079) -> (-56.7527, -69.0659) projected
  line L16 (-59.9793, -70.3529) -> (-59.9813, -73.6029) projected
  line L17 (-59.9813, -73.6029) -> (-63.2313, -73.6008) projected
  line L18 (-63.2313, -73.6008) -> (-63.2293, -70.3508) projected
  line L19 (-63.2293, -70.3508) -> (-59.9793, -70.3529) projected
  line L20 (-63.4534, -70.3067) -> (-64.6994, -73.3084) projected
  line L21 (-64.6994, -73.3084) -> (-67.7011, -72.0624) projected
  line L22 (-67.7011, -72.0624) -> (-66.455, -69.0607) projected
  line L23 (-66.455, -69.0607) -> (-63.4534, -70.3067) projected
  line L24 (-66.6438, -68.9351) -> (-68.9435, -71.2317) projected
  line L25 (-68.9435, -71.2317) -> (-71.24, -68.932) projected
  line L26 (-71.24, -68.932) -> (-68.9403, -66.6355) projected
  line L27 (-68.9403, -66.6355) -> (-66.6438, -68.9351) projected
  line L28 (-69.0665, -66.4474) -> (-72.0699, -67.6893) projected
  line L29 (-72.0699, -67.6893) -> (-73.3118, -64.686) projected
  line L30 (-73.3118, -64.686) -> (-70.3085, -63.4441) projected
  line L31 (-70.3085, -63.4441) -> (-69.0665, -66.4474) projected
  line L32 (-70.3079, -59.7483) -> (-73.3095, -58.5022) projected
  line L33 (-73.3095, -58.5022) -> (-72.0634, -55.5006) projected
  line L34 (-72.0634, -55.5006) -> (-69.0618, -56.7467) projected
  line L35 (-69.0618, -56.7467) -> (-70.3079, -59.7483) projected
  line L36 (-68.9355, -56.5569) -> (-71.2319, -54.2571) projected
  line L37 (-71.2319, -54.2571) -> (-68.932, -51.9607) projected
  line L38 (-68.932, -51.9607) -> (-66.6357, -54.2606) projected
  line L39 (-66.6357, -54.2606) -> (-68.9355, -56.5569) projected
  line L40 (-66.4458, -54.1331) -> (-67.6871, -51.1295) projected
  line L41 (-67.6871, -51.1295) -> (-64.6835, -49.8882) projected
  line L42 (-64.6835, -49.8882) -> (-63.4422, -52.8918) projected
  line L43 (-63.4422, -52.8918) -> (-66.4458, -54.1331) projected
  line L44 (-59.7474, -52.8928) -> (-58.5019, -49.891) projected
  line L45 (-58.5019, -49.891) -> (-55.5, -51.1366) projected
  line L46 (-55.5, -51.1366) -> (-56.7456, -54.1384) projected
  line L47 (-56.7456, -54.1384) -> (-59.7474, -52.8928) projected
  line L48 (-56.5557, -54.2647) -> (-54.2559, -51.9683) projected
  line L49 (-54.2559, -51.9683) -> (-51.9595, -54.2681) projected
  line L50 (-51.9595, -54.2681) -> (-54.2593, -56.5645) projected
  line L51 (-54.2593, -56.5645) -> (-56.5557, -54.2647) projected
  line L52 (-54.1334, -56.752) -> (-51.1301, -55.5101) projected
  line L53 (-51.1301, -55.5101) -> (-49.8882, -58.5135) projected
  line L54 (-49.8882, -58.5135) -> (-52.8916, -59.7554) projected
  line L55 (-52.8916, -59.7554) -> (-54.1334, -56.752) projected
  line L56 (-52.8505, -59.9795) -> (-49.6005, -59.9784) projected
  line L57 (-49.6005, -59.9784) -> (-49.5995, -63.2284) projected
  line L58 (-49.5995, -63.2284) -> (-52.8495, -63.2295) projected
  line L59 (-52.8495, -63.2295) -> (-52.8505, -59.9795) projected
  line L60 (-70.3537, -63.2194) -> (-73.6037, -63.2169) projected
  line L61 (-73.6037, -63.2169) -> (-73.6013, -59.9669) projected
  line L62 (-73.6013, -59.9669) -> (-70.3513, -59.9694) projected
  line L63 (-70.3513, -59.9694) -> (-70.3537, -63.2194) projected
  line L64 (-67.06, -63.215) -> (-67.1425, -63.2212) projected
  line L65 (-67.1425, -63.2212) -> (-67.2261, -63.2233) projected
  line L66 (-67.2261, -63.2233) -> (-67.3097, -63.2211) projected
  line L67 (-67.3097, -63.2211) -> (-67.3923, -63.2148) projected
  line L68 (-67.3923, -63.2148) -> (-67.4736, -63.2045) projected
  line L69 (-67.4736, -63.2045) -> (-67.5536, -63.1902) projected
  line L70 (-67.5536, -63.1902) -> (-67.6322, -63.172) projected
  line L71 (-67.6322, -63.172) -> (-67.7093, -63.15) projected
  line L72 (-67.7093, -63.15) -> (-67.7848, -63.1245) projected
  line L73 (-67.7848, -63.1245) -> (-67.8586, -63.0953) projected
  line L74 (-67.8586, -63.0953) -> (-67.9306, -63.0628) projected
  line L75 (-67.9306, -63.0628) -> (-68.0006, -63.0269) projected
  line L76 (-68.0006, -63.0269) -> (-68.0686, -62.9877) projected
  line L77 (-68.0686, -62.9877) -> (-68.1346, -62.9454) projected
  line L78 (-68.1346, -62.9454) -> (-68.1982, -62.9001) projected
  line L79 (-68.1982, -62.9001) -> (-68.2596, -62.8518) projected
  line L80 (-68.2596, -62.8518) -> (-68.3186, -62.8007) projected
  line L81 (-68.3186, -62.8007) -> (-68.375, -62.7469) projected
  line L82 (-68.375, -62.7469) -> (-68.4288, -62.6904) projected
  line L83 (-68.4288, -62.6904) -> (-68.4798, -62.6314) projected
  line L84 (-68.4798, -62.6314) -> (-68.528, -62.57) projected
  line L85 (-68.528, -62.57) -> (-68.5733, -62.5063) projected
  line L86 (-68.5733, -62.5063) -> (-68.6155, -62.4404) projected
  line L87 (-68.6155, -62.4404) -> (-68.6546, -62.3723) projected
  line L88 (-68.6546, -62.3723) -> (-68.6905, -62.3022) projected
  line L89 (-68.6905, -62.3022) -> (-68.723, -62.2302) projected
  line L90 (-68.723, -62.2302) -> (-68.7521, -62.1564) projected
  line L91 (-68.7521, -62.1564) -> (-68.7776, -62.0809) projected
  line L92 (-68.7776, -62.0809) -> (-68.7995, -62.0038) projected
  line L93 (-68.7995, -62.0038) -> (-68.8176, -61.9252) projected
  line L94 (-68.8176, -61.9252) -> (-68.8318, -61.8451) projected
  line L95 (-68.8318, -61.8451) -> (-68.8421, -61.7638) projected
  line L96 (-68.8421, -61.7638) -> (-68.8484, -61.6813) projected
  line L97 (-68.8484, -61.6813) -> (-68.8505, -61.5976) projected
  line L98 (-68.8505, -61.5976) -> (-68.8483, -61.514) projected
  line L99 (-68.8483, -61.514) -> (-68.842, -61.4315) projected
  line L100 (-68.842, -61.4315) -> (-68.8316, -61.3502) projected
  line L101 (-68.8316, -61.3502) -> (-68.8173, -61.2702) projected
  line L102 (-68.8173, -61.2702) -> (-68.7991, -61.1916) projected
  line L103 (-68.7991, -61.1916) -> (-68.7772, -61.1144) projected
  line L104 (-68.7772, -61.1144) -> (-68.7516, -61.039) projected
  line L105 (-68.7516, -61.039) -> (-68.7225, -60.9652) projected
  line L106 (-68.7225, -60.9652) -> (-68.6899, -60.8932) projected
  line L107 (-68.6899, -60.8932) -> (-68.654, -60.8232) projected
  line L108 (-68.654, -60.8232) -> (-68.6149, -60.7551) projected
  line L109 (-68.6149, -60.7551) -> (-68.5726, -60.6892) projected
  line L110 (-68.5726, -60.6892) -> (-68.5272, -60.6255) projected
  line L111 (-68.5272, -60.6255) -> (-68.479, -60.5641) projected
  line L112 (-68.479, -60.5641) -> (-68.4279, -60.5052) projected
  line L113 (-68.4279, -60.5052) -> (-68.374, -60.4488) projected
  line L114 (-68.374, -60.4488) -> (-68.3176, -60.395) projected
  line L115 (-68.3176, -60.395) -> (-68.2586, -60.344) projected
  line L116 (-68.2586, -60.344) -> (-68.1972, -60.2957) projected
  line L117 (-68.1972, -60.2957) -> (-68.1335, -60.2505) projected
  line L118 (-68.1335, -60.2505) -> (-68.0675, -60.2082) projected
  line L119 (-68.0675, -60.2082) -> (-67.9995, -60.1691) projected
  line L120 (-67.9995, -60.1691) -> (-67.9294, -60.1333) projected
  line L121 (-67.9294, -60.1333) -> (-67.8574, -60.1007) projected
  line L122 (-67.8574, -60.1007) -> (-67.7836, -60.0717) projected
  line L123 (-67.7836, -60.0717) -> (-67.7081, -60.0462) projected
  line L124 (-67.7081, -60.0462) -> (-67.6309, -60.0243) projected
  line L125 (-67.6309, -60.0243) -> (-67.5523, -60.0062) projected
  line L126 (-67.5523, -60.0062) -> (-67.4723, -59.9919) projected
  line L127 (-67.4723, -59.9919) -> (-67.391, -59.9816) projected
  line L128 (-67.391, -59.9816) -> (-67.3084, -59.9754) projected
  line L129 (-67.3084, -59.9754) -> (-67.2248, -59.9733) projected
  line L130 (-67.2248, -59.9733) -> (-67.1412, -59.9754) projected
  line L131 (-67.1412, -59.9754) -> (-67.0587, -59.9818) projected
  line L132 (-67.0587, -59.9818) -> (-66.9773, -59.9921) projected
  line L133 (-66.9773, -59.9921) -> (-66.8973, -60.0064) projected
  line L134 (-66.8973, -60.0064) -> (-66.8187, -60.0246) projected
  line L135 (-66.8187, -60.0246) -> (-66.7416, -60.0465) projected
  line L136 (-66.7416, -60.0465) -> (-66.6661, -60.0721) projected
  line L137 (-66.6661, -60.0721) -> (-66.5923, -60.1013) projected
  line L138 (-66.5923, -60.1013) -> (-66.5204, -60.1338) projected
  line L139 (-66.5204, -60.1338) -> (-66.4503, -60.1697) projected
  line L140 (-66.4503, -60.1697) -> (-66.3823, -60.2089) projected
  line L141 (-66.3823, -60.2089) -> (-66.3164, -60.2512) projected
  line L142 (-66.3164, -60.2512) -> (-66.2527, -60.2965) projected
  line L143 (-66.2527, -60.2965) -> (-66.1913, -60.3448) projected
  line L144 (-66.1913, -60.3448) -> (-66.1324, -60.3959) projected
  line L145 (-66.1324, -60.3959) -> (-66.0759, -60.4497) projected
  line L146 (-66.0759, -60.4497) -> (-66.0222, -60.5062) projected
  line L147 (-66.0222, -60.5062) -> (-65.9711, -60.5652) projected
  line L148 (-65.9711, -60.5652) -> (-65.9229, -60.6266) projected
  line L149 (-65.9229, -60.6266) -> (-65.8776, -60.6903) projected
  line L150 (-65.8776, -60.6903) -> (-65.8354, -60.7562) projected
  line L151 (-65.8354, -60.7562) -> (-65.7963, -60.8243) projected
  line L152 (-65.7963, -60.8243) -> (-65.7604, -60.8944) projected
  line L153 (-65.7604, -60.8944) -> (-65.7279, -60.9664) projected
  line L154 (-65.7279, -60.9664) -> (-65.6988, -61.0402) projected
  line L155 (-65.6988, -61.0402) -> (-65.6733, -61.1157) projected
  line L156 (-65.6733, -61.1157) -> (-65.6515, -61.1928) projected
  line L157 (-65.6515, -61.1928) -> (-65.6333, -61.2714) projected
  line L158 (-65.6333, -61.2714) -> (-65.6191, -61.3515) projected
  line L159 (-65.6191, -61.3515) -> (-65.6088, -61.4328) projected
  line L160 (-65.6088, -61.4328) -> (-65.6025, -61.5153) projected
  line L161 (-65.6025, -61.5153) -> (-65.6005, -61.599) projected
  line L162 (-65.6005, -61.599) -> (-65.6026, -61.6826) projected
  line L163 (-65.6026, -61.6826) -> (-65.6089, -61.7651) projected
  line L164 (-65.6089, -61.7651) -> (-65.6193, -61.8464) projected
  line L165 (-65.6193, -61.8464) -> (-65.6336, -61.9264) projected
  line L166 (-65.6336, -61.9264) -> (-65.6518, -62.005) projected
  line L167 (-65.6518, -62.005) -> (-65.6737, -62.0821) projected
  line L168 (-65.6737, -62.0821) -> (-65.6993, -62.1576) projected
  line L169 (-65.6993, -62.1576) -> (-65.7284, -62.2314) projected
  line L170 (-65.7284, -62.2314) -> (-65.761, -62.3034) projected
  line L171 (-65.761, -62.3034) -> (-65.7969, -62.3734) projected
  line L172 (-65.7969, -62.3734) -> (-65.8361, -62.4415) projected
  line L173 (-65.8361, -62.4415) -> (-65.8783, -62.5074) projected
  line L174 (-65.8783, -62.5074) -> (-65.9237, -62.5711) projected
  line L175 (-65.9237, -62.5711) -> (-65.9719, -62.6325) projected
  line L176 (-65.9719, -62.6325) -> (-66.023, -62.6914) projected
  line L177 (-66.023, -62.6914) -> (-66.0769, -62.7478) projected
  line L178 (-66.0769, -62.7478) -> (-66.1333, -62.8016) projected
  line L179 (-66.1333, -62.8016) -> (-66.1923, -62.8526) projected
  line L180 (-66.1923, -62.8526) -> (-66.2537, -62.9009) projected
  line L181 (-66.2537, -62.9009) -> (-66.3174, -62.9461) projected
  line L182 (-66.3174, -62.9461) -> (-66.3834, -62.9884) projected
  line L183 (-66.3834, -62.9884) -> (-66.4515, -63.0275) projected
  line L184 (-66.4515, -63.0275) -> (-66.5215, -63.0633) projected
  line L185 (-66.5215, -63.0633) -> (-66.5935, -63.0959) projected
  line L186 (-66.5935, -63.0959) -> (-66.6673, -63.1249) projected
  line L187 (-66.6673, -63.1249) -> (-66.7429, -63.1504) projected
  line L188 (-66.7429, -63.1504) -> (-66.82, -63.1723) projected
  line L189 (-66.82, -63.1723) -> (-66.8986, -63.1904) projected
  line L190 (-66.8986, -63.1904) -> (-66.9786, -63.2047) projected
  line L191 (-66.9786, -63.2047) -> (-67.06, -63.215) projected
  line L192 (-56.141, -59.9837) -> (-56.0584, -59.9774) projected
  line L193 (-56.0584, -59.9774) -> (-55.9748, -59.9753) projected
  line L194 (-55.9748, -59.9753) -> (-55.8912, -59.9774) projected
  line L195 (-55.8912, -59.9774) -> (-55.8087, -59.9837) projected
  line L196 (-55.8087, -59.9837) -> (-55.7273, -59.994) projected
  line L197 (-55.7273, -59.994) -> (-55.6473, -60.0083) projected
  line L198 (-55.6473, -60.0083) -> (-55.5687, -60.0265) projected
  line L199 (-55.5687, -60.0265) -> (-55.4916, -60.0484) projected
  line L200 (-55.4916, -60.0484) -> (-55.4161, -60.074) projected
  line L201 (-55.4161, -60.074) -> (-55.3423, -60.1031) projected
  line L202 (-55.3423, -60.1031) -> (-55.2703, -60.1356) projected
  line L203 (-55.2703, -60.1356) -> (-55.2003, -60.1715) projected
  line L204 (-55.2003, -60.1715) -> (-55.1322, -60.2106) projected
  line L205 (-55.1322, -60.2106) -> (-55.0663, -60.2529) projected
  line L206 (-55.0663, -60.2529) -> (-55.0026, -60.2982) projected
  line L207 (-55.0026, -60.2982) -> (-54.9412, -60.3465) projected
  line L208 (-54.9412, -60.3465) -> (-54.8822, -60.3976) projected
  line L209 (-54.8822, -60.3976) -> (-54.8258, -60.4514) projected
  line L210 (-54.8258, -60.4514) -> (-54.772, -60.5078) projected
  line L211 (-54.772, -60.5078) -> (-54.7209, -60.5668) projected
  line L212 (-54.7209, -60.5668) -> (-54.6727, -60.6282) projected
  line L213 (-54.6727, -60.6282) -> (-54.6274, -60.6919) projected
  line L214 (-54.6274, -60.6919) -> (-54.5852, -60.7578) projected
  line L215 (-54.5852, -60.7578) -> (-54.546, -60.8259) projected
  line L216 (-54.546, -60.8259) -> (-54.5102, -60.8959) projected
  line L217 (-54.5102, -60.8959) -> (-54.4776, -60.9679) projected
  line L218 (-54.4776, -60.9679) -> (-54.4485, -61.0417) projected
  line L219 (-54.4485, -61.0417) -> (-54.423, -61.1172) projected
  line L220 (-54.423, -61.1172) -> (-54.4011, -61.1944) projected
  line L221 (-54.4011, -61.1944) -> (-54.383, -61.273) projected
  line L222 (-54.383, -61.273) -> (-54.3687, -61.353) projected
  line L223 (-54.3687, -61.353) -> (-54.3584, -61.4343) projected
  line L224 (-54.3584, -61.4343) -> (-54.3521, -61.5169) projected
  line L225 (-54.3521, -61.5169) -> (-54.35, -61.6005) projected
  line L226 (-54.35, -61.6005) -> (-54.3521, -61.6841) projected
  line L227 (-54.3521, -61.6841) -> (-54.3584, -61.7666) projected
  line L228 (-54.3584, -61.7666) -> (-54.3688, -61.8479) projected
  line L229 (-54.3688, -61.8479) -> (-54.3831, -61.928) projected
  line L230 (-54.3831, -61.928) -> (-54.4012, -62.0066) projected
  line L231 (-54.4012, -62.0066) -> (-54.4231, -62.0837) projected
  line L232 (-54.4231, -62.0837) -> (-54.4487, -62.1592) projected
  line L233 (-54.4487, -62.1592) -> (-54.4778, -62.233) projected
  line L234 (-54.4778, -62.233) -> (-54.5103, -62.305) projected
  line L235 (-54.5103, -62.305) -> (-54.5462, -62.375) projected
  line L236 (-54.5462, -62.375) -> (-54.5854, -62.4431) projected
  line L237 (-54.5854, -62.4431) -> (-54.6276, -62.509) projected
  line L238 (-54.6276, -62.509) -> (-54.6729, -62.5727) projected
  line L239 (-54.6729, -62.5727) -> (-54.7212, -62.6341) projected
  line L240 (-54.7212, -62.6341) -> (-54.7723, -62.693) projected
  line L241 (-54.7723, -62.693) -> (-54.8261, -62.7495) projected
  line L242 (-54.8261, -62.7495) -> (-54.8825, -62.8033) projected
  line L243 (-54.8825, -62.8033) -> (-54.9415, -62.8543) projected
  line L244 (-54.9415, -62.8543) -> (-55.0029, -62.9026) projected
  line L245 (-55.0029, -62.9026) -> (-55.0666, -62.9479) projected
  line L246 (-55.0666, -62.9479) -> (-55.1325, -62.9901) projected
  line L247 (-55.1325, -62.9901) -> (-55.2006, -63.0292) projected
  line L248 (-55.2006, -63.0292) -> (-55.2707, -63.0651) projected
  line L249 (-55.2707, -63.0651) -> (-55.3427, -63.0977) projected
  line L250 (-55.3427, -63.0977) -> (-55.4165, -63.1267) projected
  line L251 (-55.4165, -63.1267) -> (-55.492, -63.1523) projected
  line L252 (-55.492, -63.1523) -> (-55.5691, -63.1742) projected
  line L253 (-55.5691, -63.1742) -> (-55.6477, -63.1923) projected
  line L254 (-55.6477, -63.1923) -> (-55.7277, -63.2066) projected
  line L255 (-55.7277, -63.2066) -> (-55.809, -63.2169) projected
  line L256 (-55.809, -63.2169) -> (-55.8916, -63.2232) projected
  line L257 (-55.8916, -63.2232) -> (-55.9752, -63.2253) projected
  line L258 (-55.9752, -63.2253) -> (-56.0588, -63.2232) projected
  line L259 (-56.0588, -63.2232) -> (-56.1413, -63.2169) projected
  line L260 (-56.1413, -63.2169) -> (-56.2227, -63.2065) projected
  line L261 (-56.2227, -63.2065) -> (-56.3027, -63.1922) projected
  line L262 (-56.3027, -63.1922) -> (-56.3813, -63.1741) projected
  line L263 (-56.3813, -63.1741) -> (-56.4584, -63.1522) projected
  line L264 (-56.4584, -63.1522) -> (-56.5339, -63.1266) projected
  line L265 (-56.5339, -63.1266) -> (-56.6077, -63.0975) projected
  line L266 (-56.6077, -63.0975) -> (-56.6797, -63.065) projected
  line L267 (-56.6797, -63.065) -> (-56.7497, -63.0291) projected
  line L268 (-56.7497, -63.0291) -> (-56.8178, -62.9899) projected
  line L269 (-56.8178, -62.9899) -> (-56.8837, -62.9476) projected
  line L270 (-56.8837, -62.9476) -> (-56.9474, -62.9023) projected
  line L271 (-56.9474, -62.9023) -> (-57.0088, -62.8541) projected
  line L272 (-57.0088, -62.8541) -> (-57.0678, -62.803) projected
  line L273 (-57.0678, -62.803) -> (-57.1242, -62.7492) projected
  line L274 (-57.1242, -62.7492) -> (-57.178, -62.6928) projected
  line L275 (-57.178, -62.6928) -> (-57.2291, -62.6338) projected
  line L276 (-57.2291, -62.6338) -> (-57.2773, -62.5724) projected
  line L277 (-57.2773, -62.5724) -> (-57.3226, -62.5087) projected
  line L278 (-57.3226, -62.5087) -> (-57.3648, -62.4427) projected
  line L279 (-57.3648, -62.4427) -> (-57.404, -62.3747) projected
  line L280 (-57.404, -62.3747) -> (-57.4398, -62.3046) projected
  line L281 (-57.4398, -62.3046) -> (-57.4724, -62.2326) projected
  line L282 (-57.4724, -62.2326) -> (-57.5015, -62.1588) projected
  line L283 (-57.5015, -62.1588) -> (-57.527, -62.0833) projected
  line L284 (-57.527, -62.0833) -> (-57.5489, -62.0062) projected
  line L285 (-57.5489, -62.0062) -> (-57.567, -61.9276) projected
  line L286 (-57.567, -61.9276) -> (-57.5813, -61.8476) projected
  line L287 (-57.5813, -61.8476) -> (-57.5916, -61.7662) projected
  line L288 (-57.5916, -61.7662) -> (-57.5979, -61.6837) projected
  line L289 (-57.5979, -61.6837) -> (-57.6, -61.6001) projected
  line L290 (-57.6, -61.6001) -> (-57.5979, -61.5165) projected
  line L291 (-57.5979, -61.5165) -> (-57.5916, -61.4339) projected
  line L292 (-57.5916, -61.4339) -> (-57.5812, -61.3526) projected
  line L293 (-57.5812, -61.3526) -> (-57.5669, -61.2726) projected
  line L294 (-57.5669, -61.2726) -> (-57.5488, -61.194) projected
  line L295 (-57.5488, -61.194) -> (-57.5269, -61.1169) projected
  line L296 (-57.5269, -61.1169) -> (-57.5013, -61.0414) projected
  line L297 (-57.5013, -61.0414) -> (-57.4722, -60.9676) projected